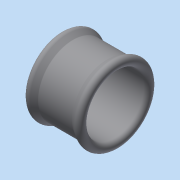
# Autodesk Inventor part: Обмотка статора
Saved by Autodesk Inventor 2016 SP1 (Build 200210100, 210)
## iProperties
Created: 2016-05-17
Part Number: Обмотка статора
Material: Медь
Document SubType Name: Modeling
Designer: a.kaluzhenin
Density: 8.94 g/cm^3
Appearance: Медь - сатинированная
Mass: 4741.25 g
Surface Area: 987.962 cm^2
Volume: 530.341 cm^3
Author: a.kaluzhenin
Autodesk Inventor part; units mm, degrees
ref_plane "YZ Plane" through (0, 0, 0) normal (1, 0, 0) x (0, 1, 0)
ref_plane "XZ Plane" through (0, 0, 0) normal (0, 1, 0) x (-1, 0, 0)
ref_plane "XY Plane" through (0, 0, 0) normal (0, 0, 1) x (1, 0, 0)
sketch "Эскиз1" plane through (0, 0, 0) normal (0, 0, 1) x (1, 0, 0)
  line L0 (-32.4641, 68) -> (32.4641, 68)
  line L1 (-47, 57.6012) -> (47, 57.6012)
  line L2 (33.4641, 68.2679) -> (43, 73.7735)
  arc A0 (47, 57.6012) -> (43, 73.7735) centre (47, 66.182) ccw
  line L3 (0, 57.6012) -> (0, 68) construction
  line L4 (-33.4641, 68.2679) -> (-43, 73.7735)
  arc A1 (-43, 73.7735) -> (-47, 57.6012) centre (-47, 66.182) ccw
  arc A2 (-33.4641, 68.2679) -> (-32.4641, 68) centre (-32.4641, 70) ccw
  arc A3 (32.4641, 68) -> (33.4641, 68.2679) centre (32.4641, 70) ccw
  line L5 (-80.3461, 0) -> (80.3461, 0) projected
  point P0 (0, 0)
  point P1 (0, 57.6012)
  point P2 (0, 68)
  point P3 (-33, 68)
  point P4 (33, 68)
  point P5 (55.5782, 66.3924)
  dimension "d0" = 66
  dimension "d1" = 94
  dimension "d2" = 30
  dimension "d3" = 10
  dimension "d4" = 2
  dimension "d5" = 2
  constraints: 10 end point, 9 point on circle, 4 centre point, 4 point on line, 4 tangent, 2 coincident, 2 horizontal, 2 midpoint, 2 symmetric about line, 1 perpendicular, 1 vertical alignment, 1 other
  measures "d0" distance of point (33, 68) point (-33, 68)
  measures "d1" distance of L1.start L1.end
  measures "d2" angle of L2 L0
  measures "d3" horizontal distance of L2.end point (33, 68)
  measures "d4" radius of A2
  measures "d5" radius of A3
revolve "Вращение1" add sketch "Эскиз1" angle 360 about axis through (-10, 0, 0) along (1, 0, 0)
